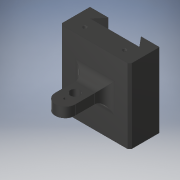
# Autodesk Inventor part: BT401_trajan20_21
Saved by Autodesk Inventor 2022.2 (Build 262287000, 287)
## iProperties
Company: HTBLA Kaindorf
RuleStatus: InUse
Created: 2022-08-07
Part Number: BT401_trajan20_21
Project: Zeichenmaschine_v2
Material: Kunststoff, undurchsichtig Schwarz
Description: Stifthalter außen
Document SubType Name: Modeling
Designer: trajan20
Density: 0.952 g/cm^3
Appearance: Glatt - Schwarz
Mass: 127.546 g
Surface Area: 240.551 cm^2
Volume: 133.976 cm^3
AfterDocNew0: iProperties-Editor_aufrufen
Author: jan
Keywords: 2021
Autodesk Inventor part; units mm, degrees
ref_plane "YZ Plane" through (0, 0, 0) normal (1, 0, 0) x (0, 1, 0)
ref_plane "XZ Plane" through (0, 0, 0) normal (0, 1, 0) x (-1, 0, 0)
ref_plane "XY Plane" through (0, 0, 0) normal (0, 0, 1) x (1, 0, 0)
sketch "Skizze3" plane through (0, 0, 0) normal (0, 0, 1) x (1, 0, 0)
  circle A0 centre (0, 0) radius 5
  circle A1 centre (10, 0) radius 1.5
  line L0 (0, -49) -> (0, 49) projected
  line L1 (-64, 0) -> (34, 0) projected
  arc A2 (10, -10) -> (10, 10) centre (10, 0) ccw
  line L2 (10, -10) -> (0, -10)
  line L3 (10, 10) -> (0, 10)
  arc A3 (0, 10) -> (0, -10) centre (0, 0) ccw
  line L4 (0, -10) -> (-20, -10)
  line L5 (0, 10) -> (-20, 10)
  line L6 (-20, -10) -> (-20, -35)
  line L7 (-20, -35) -> (-50, -35)
  line L8 (-50, -35) -> (-50, 35)
  line L9 (-50, 35) -> (-20, 35)
  line L10 (-20, 35) -> (-20, 10)
  line L11 (-50, -16.609) -> (-40, -25)
  line L12 (-40, -25) -> (-40, 25)
  line L13 (-40, 25) -> (-50, 16.609)
  line L14 (-20, -10) -> (-20, 10)
  point P0 (-10, 0)
  dimension "d5" = 10
  dimension "d6" = 3
  dimension "d7" = 10
  dimension "d8" = 20
  dimension "d10" = 10
  dimension "d11" = 50
  dimension "d12" = 30
  dimension "d13" = 20
  dimension "d15" = 25
  dimension "d16" = 25
  dimension "d17" = 10
  dimension "d19" = 50
  constraints: 26 end point, 6 point on line, 5 perpendicular, 4 centre point, 4 point on circle, 3 coincident, 3 tangent, 2 horizontal, 1 parallel, 1 vertical, 1 other
  measures "d5" diameter of A0
  measures "d6" diameter of A1
  measures "d7" distance from line of L0 A1.centre
  measures "d8" diameter of A2
  measures "d10" radius of A3
  measures "d11" angle of L8 L11
  measures "d12" distance between parallel lines of L8 L6
  measures "d13" distance of L2.end L4.end
  measures "d15" distance between parallel lines of L7 L4
  measures "d16" distance between parallel lines of L9 L5
  measures "d17" distance between parallel lines of L8 L12
  measures "d19" distance of L11.end L12.end
extrude "Extrusion3" add sketch "Skizze3" along normal mid plane 10 contours L1 A1 A2 L2 L0 A0 | A0 L0 L3 A2 L1 A1 | A0 L1 A3 L0 | L0 A3 L1 A0 | A3 L1 L14 L5 | L4 L14 L1 A3
extrude "Extrusion4" add sketch "Skizze3" along normal mid plane 75 contours L14 L1 L12 L13 L8 L9 L10 | L6 L7 L8 L11 L12 L1 L14
chamfer "Fase1" distance 2 angle 45 2 edges at (-20, 35, 0) (-20, -35, 0)
fillet "Rundung1" radius 10 4 edges at (-20, 0, 5) (-20, -10, 0) (-20, 0, -5) (-20, 10, 0)
sketch "Skizze5" plane through (0, 0, 37.5) normal (0, 0, 1) x (1, 0, 0)
  line L0 (-50, -35) -> (-22, -35) projected
  line L1 (-20, -33) -> (-20, 33) projected
  line L2 (-22, 35) -> (-50, 35) projected
  point P0 (0, 0)
  point P1 (-30, 20)
  point P2 (-30, -20)
  dimension "d30" = 15
  dimension "d31" = 10
  dimension "d32" = 15
  dimension "d33" = 10
  measures "d30" distance from line of L0 point (-30, -20)
  measures "d31" distance from line of L1 point (-30, -20)
  measures "d32" distance from line of L2 point (-30, 20)
  measures "d33" distance from line of L1 point (-30, 20)
hole "Bohrung1" at (-30, 20, 37.5) at (-30, -20, 37.5) direction (0, 0, -1) diameter 4.134 depth 15 thread size "M5x0.8" class "6H" standard "ISO Metric profile"
